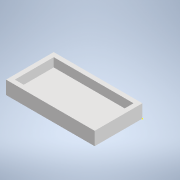
# Autodesk Inventor part: box final
Saved by Autodesk Inventor 2022 (Build 260153000, 153)
## iProperties
Created: 2022-05-06
Part Number: box final
Material: Generic
Document SubType Name: Modeling
Designer: Asus
Density: 1 g/cm^3
Appearance: Default
Author: Asus
Autodesk Inventor part; units mm, degrees
ref_plane "YZ Plane" through (0, 0, 0) normal (1, 0, 0) x (0, 1, 0)
ref_plane "XZ Plane" through (0, 0, 0) normal (0, 1, 0) x (-1, 0, 0)
ref_plane "XY Plane" through (0, 0, 0) normal (0, 0, 1) x (1, 0, 0)
sketch "Sketch1" plane through (0, 0, 0) normal (0, 1, 0) x (-1, 0, 0)
  line L0 (-0.0288, 0) -> (253.9712, 0)
  line L1 (253.9712, 0) -> (253.9712, 136.7472)
  line L2 (253.9712, 136.7472) -> (-0.0288, 136.7472)
  line L3 (-0.0288, 136.7472) -> (-0.0288, 0)
  line L4 (253.9712, 136.7472) -> (-0.0288, 136.7472)
  line L5 (-0.0288, 136.7472) -> (-0.0288, 0)
  line L6 (-0.0288, 0) -> (253.9712, 0)
  line L7 (253.9712, 0) -> (253.9712, 136.7472)
  line L8 (-0.0288, 136.7472) -> (253.9712, 136.7472)
  line L9 (253.9712, 136.7472) -> (253.9712, 0)
  line L10 (253.9712, 0) -> (-0.0288, 0)
  line L11 (-0.0288, 0) -> (-0.0288, 136.7472)
  dimension "d0" = 254
  dimension "d1" = 136.7536
  constraints: 24 end point, 6 parallel, 3 horizontal, 3 perpendicular
  measures "d0" distance of L2.end L1.end
extrude "Extrusion1" add sketch "Sketch1" along normal blind 38.1
shell "Shell1" thickness 12.7 removed faces 1 at (-169.3045, 38.1, 45.5824)
sketch "Sketch2" plane through (-241.2712, 12.7, 124.0472) normal (0, 1, 0) x (1, 0, 0)
  circle A0 centre (17.0726, 213.7662) radius 0.7982
  point P0 (241.2712, 124.0472)
  constraints: 1 centre point
extrude "Extrusion2" add sketch "Sketch2" along normal blind 0.254
sketch "Sketch3" plane through (-224.1986, 12.954, -89.719) normal (0, 1, 0) x (1, 0, 0)
  point P0 (224.1986, -89.719)
  point P1 (-0.0033, -0.0074)
hole "Hole1" at (-224.2019, 12.954, -89.7115) direction (0, -1, 0) diameter 1.6002 end through all
shell "Shell2" [suppressed]
sketch "Sketch4" plane through (0, 0, 0) normal (0, -1, 0) x (1, 0, 0)
  point P0 (0, 0)
body "Solid1"
